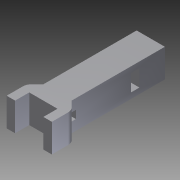
# Autodesk Inventor part: proteccionQuadCopter
Saved by Autodesk Inventor 2012 (Build 160160000, 160)
## iProperties
Created: 2013-01-10
Part Number: proteccionQuadCopter
Material: Default
Document SubType Name: Modeling
Designer: Pablo
Density: 1 g/cm^3
Author: Pablo
Autodesk Inventor part; units mm, degrees
ref_plane "YZ Plane" through (0, 0, 0) normal (1, 0, 0) x (0, 1, 0)
ref_plane "XZ Plane" through (0, 0, 0) normal (0, 1, 0) x (-1, 0, 0)
ref_plane "XY Plane" through (0, 0, 0) normal (0, 0, 1) x (1, 0, 0)
sketch "Boceto1" plane through (0, 0, 0) normal (0, 0, 1) x (1, 0, 0)
  line L0 (0, 0) -> (3, 0)
  line L1 (3, 0) -> (3, 5)
  line L2 (3, 5) -> (13, 5)
  line L3 (13, 5) -> (13, 0)
  line L4 (13, 0) -> (16, 0)
  line L5 (16, 0) -> (16, 8)
  line L6 (0, 0) -> (0, 8)
  line L7 (8, 5) -> (8, 8)
  line L8 (8, 8) -> (4.5, 8)
  line L9 (8, 8) -> (11.5, 8)
  line L10 (11.5, 8) -> (11.5, 43)
  line L11 (11.5, 43) -> (4.5, 43)
  line L12 (4.5, 43) -> (4.5, 8)
  line L13 (0, 8) -> (4.5, 8)
  line L14 (11.5, 8) -> (16, 8)
  dimension "d0" = 3
  dimension "d1" = 5
  dimension "d2" = 10
  dimension "d3" = 3
  dimension "d4" = 8
  dimension "d5" = 8
  dimension "d6" = 3
  dimension "d7" = 3.5
  dimension "d8" = 3.5
  dimension "d9" = 35
  dimension "d10" = 7
  constraints: 30 end point, 6 perpendicular, 4 parallel, 2 collinear, 1 horizontal, 1 midpoint
  measures "d0" distance of L0.start L0.end
  measures "d1" distance of L0.end L1.end
  measures "d2" distance of L1.end L2.end
  measures "d3" distance of L3.end L4.end
  measures "d4" distance of L4.end L5.end
  measures "d5" distance of L0.start L6.end
  measures "d6" distance of L7.start L7.end
  measures "d7" distance of L7.end L8.end
  measures "d8" distance of L7.end L9.end
  measures "d9" distance of L9.end L10.end
  measures "d10" distance of L10.end L11.end
extrude "Extrusión1" add sketch "Boceto1" along normal blind 10
sketch "Boceto2" plane through (11.5, 8, 0) normal (1, 0, 0) x (0, 0, -1)
  line L0 (-10, 35) -> (-10, 0) projected
  line L1 (0, 0) -> (-10, 0) projected
  line L2 (0, 0) -> (0, 35) projected
  line L3 (0, 35) -> (-10, 35) projected
  line L4 (-10, 35) -> (-10, 26)
  line L5 (0, 35) -> (-10, 35)
  line L6 (0, 35) -> (0, 26)
  line L7 (0, 26) -> (-10, 26)
  line L8 (-5, 26) -> (-2, 26)
  line L9 (-2, 26) -> (-2, 23)
  line L10 (-2, 23) -> (-8, 23)
  line L11 (-8, 23) -> (-8, 26)
  point P0 (0, -8)
  dimension "d13" = 9
  dimension "d14" = 9
  dimension "d15" = 3
  dimension "d16" = 3
  dimension "d17" = 6
  constraints: 16 end point, 4 point on line, 2 perpendicular, 1 collinear, 1 midpoint, 1 parallel
  measures "d13" distance of L0.start L4.end
  measures "d14" distance of L2.end L6.end
  measures "d15" distance of L8.start L8.end
  measures "d16" distance of L8.end L9.end
  measures "d17" distance of L9.end L10.end
sketch "Boceto3" plane through (4.5, 43, 0) normal (0, 1, 0) x (1, 0, 0)
  circle A0 centre (3.5, -5) radius 1.6
  point P0 (-4.5, 0)
  dimension "d18" = 3.2
  constraints: 1 centre point
  measures "d18" diameter of A0
extrude "Extrusión2" cut sketch "Boceto3" against normal blind 9
extrude "Extrusión3" add sketch "Boceto2" along normal blind 1.5 contours L3 L2 L7 L0 | L7 L11 L10 L9 L2 L1 L0
sketch "Boceto4" plane through (4.5, 8, 0) normal (-1, 0, 0) x (0, 0, 1)
  line L0 (10, 0) -> (10, 35) projected
  line L1 (0, 35) -> (10, 35) projected
  line L2 (0, 35) -> (0, 0) projected
  line L3 (10, 0) -> (0, 0) projected
  point P0 (0, -8)
extrude "Extrusión4" add sketch "Boceto4" along normal blind 1.5
sketch "Boceto5" plane through (11.5, 31, 8) normal (1, 0, 0) x (0, 0, -1)
  line L0 (0, 3) -> (0, 0) projected
  line L1 (0, 0) -> (6, 0) projected
  line L2 (6, 0) -> (6, 3) projected
  line L3 (6, 3) -> (0, 3) projected
  point P0 (8, -31)
extrude "Extrusión5" cut sketch "Boceto5" against normal blind 7
chamfer "Chaflán1" distance 2 angle 45 1 edges at (13, 8, 5)
fillet "Empalme1" radius 3 1 edges at (16, 8, 5)
chamfer "Chaflán2" distance 2 angle 45 1 edges at (3, 8, 5)
fillet "Empalme2" radius 3 1 edges at (0, 8, 5)
sketch "Boceto6" plane through (13, 8, 0) normal (1, 0, 0) x (0, 0, -1)
  line L0 (0, 2) -> (-10, 2) projected
  line L1 (-5, 2) -> (-3.6, 2)
  line L2 (-3.6, 2) -> (-6.4, 2)
  line L3 (-6.4, 2) -> (-6.4, 3.5)
  line L4 (-6.4, 3.5) -> (-3.6, 3.5)
  line L5 (-3.6, 3.5) -> (-3.6, 2)
  point P0 (0, -8)
  dimension "d35" = 1.4
  dimension "d36" = 2.8
  dimension "d37" = 1.5
  constraints: 10 end point, 2 perpendicular, 2 point on line, 1 midpoint, 1 parallel
  measures "d35" distance of L1.start L1.end
  measures "d36" distance of L1.end L2.end
  measures "d37" distance of L2.end L3.end
extrude "Extrusión6" cut sketch "Boceto6" against normal blind 20
